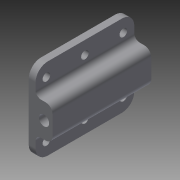
# Autodesk Inventor part: top axle holder 2
Saved by Autodesk Inventor 2015 (Build 190159000, 159)
## iProperties
Created: 2014-11-02
Part Number: top axle holder 2
Material: Generic
Document SubType Name: Modeling
Designer: jesse
Density: 1 g/cm^3
Appearance: Default
Author: jesse
Autodesk Inventor part; units mm, degrees
ref_plane "YZ Plane" through (0, 0, 0) normal (1, 0, 0) x (0, 1, 0)
ref_plane "XZ Plane" through (0, 0, 0) normal (0, 1, 0) x (-1, 0, 0)
ref_plane "XY Plane" through (0, 0, 0) normal (0, 0, 1) x (1, 0, 0)
sketch "Sketch1" plane through (0, 0, 0) normal (1, 0, 0) x (0, 1, 0)
  line L0 (0, 0) -> (38.1, 0)
  line L1 (38.1, 0) -> (38.1, -46.101)
  line L2 (38.1, -46.101) -> (0, -46.101)
  line L3 (0, -46.101) -> (0, 0)
  dimension "d0" = 38.1
  dimension "d1" = 46.101
  constraints: 8 end point, 2 parallel, 1 horizontal, 1 perpendicular
  measures "d0" distance of L1.end L2.end
  measures "d1" distance of L0.end L1.end
extrude "Extrusion1" add sketch "Sketch1" along normal blind 3.175
sketch "Sketch2" plane through (3.175, 0, 0) normal (1, 0, 0) x (0, 0, -1)
  line L0 (0, 38.1) -> (0, 0) construction
  line L1 (0, 0) -> (46.101, 0) construction
  line L2 (46.101, 0) -> (46.101, 38.1) construction
  line L3 (46.101, 38.1) -> (0, 38.1) construction
  line L4 (0, 38.1) -> (0, 0) construction
  line L5 (0, 19.05) -> (46.101, 19.05) construction
  line L6 (46.101, 38.1) -> (0, 38.1) construction
  line L7 (0, 0) -> (46.101, 0) construction
  line L8 (46.101, 0) -> (46.101, 38.1) projected
  line L9 (23.0505, 19.05) -> (23.0505, 6.0641) construction
  line L10 (23.0505, 19.05) -> (23.0505, 32.0359) construction
  line L11 (17.0623, 6.0641) -> (23.0505, 6.0641) construction
  line L12 (23.0505, 6.0641) -> (29.0387, 6.0641) construction
  line L13 (17.0623, 6.0641) -> (17.0623, 7.2131) construction
  line L14 (29.0387, 6.0641) -> (29.0387, 7.2131) construction
  line L15 (29.0387, 6.0641) -> (35.0269, 6.0641) construction
  line L16 (35.0269, 6.0641) -> (41.0151, 6.0641) construction
  line L17 (41.0151, 6.0641) -> (41.0151, 7.2131) construction
  line L18 (17.0623, 6.0641) -> (11.0741, 6.0641) construction
  line L19 (11.0741, 6.0641) -> (5.0859, 6.0641) construction
  line L20 (5.0859, 7.2131) -> (5.0859, 6.0641) construction
  circle A0 centre (23.0505, 6.0641) radius 1.7859
  circle A1 centre (5.0859, 6.0641) radius 1.7859
  circle A2 centre (41.0151, 6.0641) radius 1.7859
  line L21 (5.0859, 6.0641) -> (5.0859, 32.0359) construction
  line L22 (5.0859, 32.0359) -> (23.0505, 32.0359) construction
  line L23 (23.0505, 32.0359) -> (41.0151, 32.0359) construction
  line L24 (41.0151, 32.0359) -> (41.0151, 6.0641) construction
  circle A3 centre (5.0859, 32.0359) radius 1.7859
  circle A4 centre (23.0505, 32.0359) radius 1.7859
  circle A5 centre (41.0151, 32.0359) radius 1.7859
  dimension "d16" = 3.5719
  constraints: 34 end point, 7 collinear, 6 centre point, 6 coincident, 5 equal radius, 4 horizontal, 4 point on line, 4 vertical, 3 midpoint, 3 perpendicular
  measures "d16" diameter of A0
extrude "Extrusion2" cut sketch "Sketch2" against normal through all
sketch "Sketch3" plane through (3.175, 0, 0) normal (1, 0, 0) x (0, 0, -1)
  line L0 (0, 38.1) -> (0, 0) projected
  line L1 (0, 19.05) -> (46.101, 19.05)
  line L2 (46.101, 0) -> (46.101, 38.1) projected
  line L3 (0, 11.3401) -> (46.101, 11.3401)
  line L4 (46.101, 11.3401) -> (46.101, 26.7599)
  line L5 (46.101, 26.7599) -> (0, 26.7599)
  line L6 (0, 26.7599) -> (0, 11.3401)
  line L7 (0, 11.3401) -> (46.101, 26.7599) construction
  line L8 (46.101, 11.3401) -> (0, 26.7599) construction
  point P0 (23.0505, 19.05)
  constraints: 14 end point, 5 midpoint, 2 parallel, 1 horizontal, 1 perpendicular, 1 point on line
extrude "Extrusion3" add sketch "Sketch3" along normal blind 7.9375
sketch "Sketch4" plane through (0, 0, 0) normal (0, 0, 1) x (1, 0, 0)
  line L0 (0, 0) -> (0, 38.1) projected
  line L1 (0, 0) -> (3.175, 0) projected
  line L2 (3.175, 11.3401) -> (3.175, 0) projected
  line L3 (3.175, 11.3401) -> (11.1125, 11.3401) projected
  line L4 (11.1125, 26.7599) -> (11.1125, 11.3401) projected
  line L5 (3.175, 26.7599) -> (11.1125, 26.7599) projected
  line L6 (3.175, 38.1) -> (3.175, 26.7599) projected
  line L7 (0, 38.1) -> (3.175, 38.1) projected
  line L8 (3.175, 26.7599) -> (3.175, 11.3401)
  line L9 (11.1125, 19.05) -> (3.175, 19.05) construction
  line L10 (3.175, 26.7599) -> (11.1125, 26.7599) construction
  line L11 (7.1437, 26.7599) -> (7.1438, 11.3401) construction
  circle A0 centre (7.1438, 19.05) radius 2.3876
  dimension "d9" = 4.7752
  constraints: 6 end point, 5 midpoint, 1 centre point, 1 vertical
  measures "d9" diameter of A0
extrude "Extrusion4" cut sketch "Sketch4" against normal through all contours A0
fillet "Fillet1" radius 3.175 2 edges at (11.1125, 26.7599, -23.0505) (11.1125, 11.3401, -23.0505)
fillet "Fillet2" radius 2.54 2 edges at (3.175, 26.7599, -23.0505) (3.175, 11.3401, -23.0505)
fillet "Fillet4" radius 5.715 4 edges at (1.5875, 0, -46.101) (1.5875, 0, 0) (1.5875, 38.1, 0) (1.5875, 38.1, -46.101)
body "Solid1"
